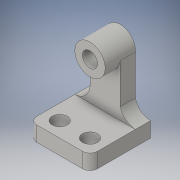
# Autodesk Inventor part: Part1
Saved by Autodesk Inventor 2016 (Build 200138000, 138)
## iProperties
Created: 2017-03-03
Part Number: Part1
Material: Generic
Document SubType Name: Modeling
Designer: 170007
Density: 1 g/cm^3
Appearance: Default
Author: 170007
Autodesk Inventor part; units mm, degrees
ref_plane "YZ Plane" through (0, 0, 0) normal (1, 0, 0) x (0, 1, 0)
ref_plane "XZ Plane" through (0, 0, 0) normal (0, 1, 0) x (-1, 0, 0)
ref_plane "XY Plane" through (0, 0, 0) normal (0, 0, 1) x (1, 0, 0)
sketch "Sketch1" plane through (0, 0, 0) normal (0, 1, 0) x (-1, 0, 0)
  line L0 (0, 0) -> (50.8, 0)
  line L1 (50.8, 0) -> (50.8, -38.1)
  line L2 (50.8, -38.1) -> (0, -38.1)
  line L3 (0, -38.1) -> (0, 0)
  dimension "d0" = 50.8
  dimension "d1" = 38.1
  constraints: 8 end point, 2 parallel, 1 horizontal, 1 perpendicular
  measures "d0" distance of L1.end L2.end
  measures "d1" distance of L0.end L1.end
extrude "Extrusion1" add sketch "Sketch1" along normal blind 12.7
fillet "Fillet1" radius 6.35 2 edges at (0, 6.35, 0) (-50.8, 6.35, 0)
sketch "Sketch2" plane through (0, 12.7, 0) normal (0, 1, 0) x (1, 0, 0)
  circle A0 centre (-12.7, 12.7) radius 6.35
  circle A1 centre (-38.1, 12.7) radius 6.35
  line L0 (-50.8, 38.1) -> (-50.8, 6.35) projected
  line L1 (-44.45, 0) -> (-6.35, 0) projected
  point P0 (0, 0)
  dimension "d5" = 12.7
  dimension "d6" = 12.7
  dimension "d7" = 12.7
  dimension "d8" = 12.7
  constraints: 2 centre point
  measures "d5" diameter of A0
  measures "d6" diameter of A1
  measures "d7" distance from line of A1.centre L0
  measures "d8" distance from line of A1.centre L1
extrude "Extrusion2" cut sketch "Sketch2" against normal blind 12.7
sketch "Sketch3" plane through (0, 0, -38.1) normal (0, 0, -1) x (-1, 0, 0)
  line L0 (6.35, 0) -> (0, 0) projected
  line L1 (0, 0) -> (50.8, 0)
  line L2 (50.8, 0) -> (50.8, 57.15)
  line L3 (50.8, 57.15) -> (0, 57.15)
  line L4 (0, 57.15) -> (0, 0)
  dimension "d11" = 57.15
  constraints: 8 end point, 2 parallel, 1 horizontal, 1 perpendicular
  measures "d11" distance of L2.end L1.end
extrude "Extrusion3" add sketch "Sketch3" along normal blind 12.7
sketch "Sketch4" plane through (0, 0, -38.1) normal (0, 0, 1) x (1, 0, 0)
  line L0 (0, 57.15) -> (0, 12.7) projected
  line L1 (0, 57.15) -> (-12.7, 57.15)
  line L2 (-12.7, 57.15) -> (-12.7, 12.7)
  line L3 (-12.7, 12.7) -> (0, 12.7)
  line L4 (0, 12.7) -> (0, 57.15)
  line L5 (-50.8, 12.7) -> (-44.45, 12.7) projected
  line L6 (-50.8, 57.15) -> (0, 57.15) projected
  line L7 (-50.8, 12.7) -> (-38.1, 12.7)
  line L8 (-38.1, 12.7) -> (-38.1, 57.15)
  line L9 (-38.1, 57.15) -> (-50.8, 57.15)
  line L10 (-50.8, 57.15) -> (-50.8, 12.7)
  point P0 (0, 0)
  dimension "d14" = 12.7
  dimension "d15" = 12.7
  constraints: 16 end point, 4 parallel, 2 horizontal, 2 perpendicular, 1 point on line
  measures "d14" distance between parallel lines of L0 L2
  measures "d15" distance of L9.end L8.end
sketch "Sketch5" plane through (0, 0, -38.1) normal (0, 0, 1) x (1, 0, 0)
  line L0 (-50.8, 57.15) -> (0, 57.15) projected
  line L1 (-38.0673, 57.15) -> (-38.0673, 24.8104)
  line L2 (0, 12.7) -> (-50.8, 12.7) projected
  arc A0 (-50.8, 12.7) -> (-38.0673, 24.8104) centre (-51.1401, 25.8062) ccw
  line L3 (-12.7393, 57.15) -> (-12.7393, 22.9207)
  arc A1 (-12.7393, 22.9207) -> (0, 12.7) centre (0.0454, 25.8063) ccw
  line L4 (-38.0673, 57.15) -> (-50.8, 57.15)
  line L5 (-50.8, 12.7) -> (-50.8, 57.15) projected
  line L6 (-50.8, 12.7) -> (-50.8, 57.15)
  line L7 (-12.7393, 57.15) -> (0, 57.15)
  line L8 (0, 57.15) -> (0, 12.7) projected
  line L9 (0, 57.15) -> (0, 12.7)
  point P0 (0, 0)
  dimension "d16" = 13.1064
  constraints: 12 end point, 4 collinear, 4 point on circle, 2 centre point, 2 point on line, 2 vertical
  measures "d16" radius of A1
extrude "Extrusion4" cut sketch "Sketch5" against normal blind 33.3375 contours L0 L1 A0 L5 | L0 L8 A1 L3
sketch "Sketch6" plane through (0, 0, -50.8) normal (0, 0, -1) x (-1, 0, 0)
  line L0 (38.0673, 57.15) -> (12.7393, 57.15) projected
  circle A0 centre (25.4033, 57.15) radius 12.7
  point P0 (0, 0)
  dimension "d19" = 25.4
  constraints: 1 centre point, 1 midpoint
  measures "d19" diameter of A0
extrude "Extrusion5" add sketch "Sketch6" against normal blind 25.4
sketch "Sketch7" plane through (-25.4033, 57.15, -25.4) normal (0, 0, 1) x (1, 0, 0)
  circle A0 centre (0, 0) radius 6.35
  point P0 (25.4033, -57.15)
  dimension "d22" = 12.7
  constraints: 1 centre point
  measures "d22" diameter of A0
extrude "Extrusion6" cut sketch "Sketch7" against normal blind 2540
body "Solid1"
